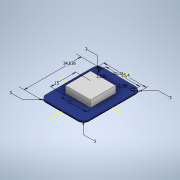
# Autodesk Inventor part: GPSSensor
Saved by Autodesk Inventor 2021 (Build 250183000, 183)
## iProperties
Created: 2020-12-16
Part Number: GPSSensor
Material: Generisch
Document SubType Name: Modeling
Designer: laure
Density: 1 g/cm^3
Appearance: Vorgabe
Author: laure
Autodesk Inventor part; units mm, degrees
ref_plane "YZ Plane" through (0, 0, 0) normal (1, 0, 0) x (0, 1, 0)
ref_plane "XZ Plane" through (0, 0, 0) normal (0, 1, 0) x (-1, 0, 0)
ref_plane "XY Plane" through (0, 0, 0) normal (0, 0, 1) x (1, 0, 0)
sketch "Skizze1" plane through (0, 0, 0) normal (0, 1, 0) x (-1, 0, 0)
  line L0 (9.7, -17.018) -> (-9.7, -17.018)
  line L1 (-12.7, -14.018) -> (-12.7, 14.018)
  line L2 (-9.7, 17.018) -> (9.7, 17.018)
  line L3 (12.7, 14.018) -> (12.7, -14.018)
  line L4 (0, -24.695) -> (0, 24.695) projected
  line L5 (18.6498, 0) -> (-18.6498, 0) projected
  circle A0 centre (10.16, -14.9291) radius 1.143
  circle A1 centre (-10.16, -14.9291) radius 1.143
  arc A2 (9.7, -17.018) -> (12.7, -14.018) centre (9.7, -14.018) ccw
  arc A3 (-12.7, -14.018) -> (-9.7, -17.018) centre (-9.7, -14.018) ccw
  arc A4 (12.7, 14.018) -> (9.7, 17.018) centre (9.7, 14.018) ccw
  arc A5 (-9.7, 17.018) -> (-12.7, 14.018) centre (-9.7, 14.018) ccw
  line L6 (7.5, -7.5) -> (-7.5, -7.5)
  line L7 (-7.5, -7.5) -> (-7.5, 7.5)
  line L8 (-7.5, 7.5) -> (7.5, 7.5)
  line L9 (7.5, 7.5) -> (7.5, -7.5)
  point P0 (0, 0)
  dimension "d0" = 25.4
  dimension "d1" = 34.036
  dimension "d2" = 2.286
  dimension "d3" = 2.286
  dimension "d4" = 20.32
  dimension "d5" = 3
  dimension "d6" = 3
  dimension "d7" = 3
  dimension "d8" = 3
  dimension "d9" = 15
  dimension "d10" = 15
  constraints: 16 end point, 8 point on circle, 8 tangent, 6 centre point, 4 parallel, 2 horizontal, 2 perpendicular, 1 symmetric about line, 4 other
  measures "d0" distance between parallel lines of L1 L3
  measures "d1" distance between parallel lines of L0 L2
  measures "d2" diameter of A0
  measures "d3" diameter of A1
  measures "d4" distance of A1.centre A0.centre
  measures "d5" radius of A2
  measures "d6" radius of A3
  measures "d7" radius of A4
  measures "d8" radius of A5
  measures "d9" distance between parallel lines of L8 L6
  measures "d10" distance between parallel lines of L7 L9
extrude "Extrusion1" add sketch "Skizze1" along normal blind 1
extrude "Extrusion2" add sketch "Skizze1" along normal blind 5 contours L6 L7 L5 L4 | L4 L5 L9 L6 | L5 L7 L8 L4 | L4 L8 L9 L5
